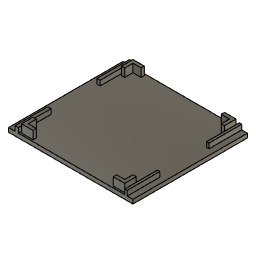
Batterystand V4 (Autodesk Fusion 360 design; units mm, degrees)
Autodesk Fusion 360 part; units mm, degrees
sketch "Sketch2" plane through (0, 0, 0) normal (0, 0, 1) x (1, 0, 0)
  line L0 (0, 0) -> (76, 0)
  line L1 (76, 0) -> (76, 70)
  line L2 (76, 70) -> (0, 70)
  line L3 (0, 70) -> (0, 0)
  dimension "d20" = 76
  dimension "d21" = 70
  constraint horizontal L0
  constraint vertical L1
  constraint horizontal L2
  constraint vertical L3
  constraint coincident L0.start L3.end
  measures "d20" distance of L0.start L0.end
  measures "d21" distance of L0.start L2.end
extrude "Extrude1" add sketch "Sketch2" along normal blind 2.9
sketch "Sketch3" plane through (0, 0, 2.9) normal (0, 0, 1) x (-1, 0, 0)
  line L0 (0, -70) -> (0, 0)
  line L1 (0, 0) -> (-76, 0)
  line L2 (-76, 0) -> (-76, -70)
  line L3 (-76, -70) -> (0, -70)
  line L4 (0, -70) -> (-7, -70)
  line L5 (-7, -70) -> (-7, -69)
  line L6 (-7, -69) -> (-14, -69)
  line L7 (-14, -69) -> (-14, -67)
  line L8 (-14, -67) -> (-9, -67)
  line L9 (-9, -67) -> (-9, -62)
  line L10 (-9, -62) -> (-7, -62)
  line L11 (-7, -62) -> (-7, -69)
  line L12 (-9, -67) -> (-68, -67)
  line L13 (-68, -67) -> (-63, -67)
  line L14 (-63, -67) -> (-63, -69)
  line L15 (-63, -69) -> (-70, -69)
  line L16 (-70, -69) -> (-70, -62)
  line L17 (-70, -62) -> (-68, -62)
  line L18 (-68, -62) -> (-68, -67)
  line L19 (-68, -67) -> (-68, -3)
  line L20 (-68, -3) -> (-63, -3)
  line L21 (-63, -3) -> (-63, -1)
  line L22 (-63, -1) -> (-70, -1)
  line L23 (-70, -1) -> (-70, -8)
  line L24 (-70, -8) -> (-68, -8)
  line L25 (-68, -3) -> (-68, -8)
  line L26 (-9, -67) -> (-9, -3)
  line L27 (-9, -3) -> (-14, -3)
  line L28 (-14, -3) -> (-14, -1)
  line L29 (-14, -1) -> (-7, -1)
  line L30 (-7, -1) -> (-7, -8)
  line L31 (-7, -8) -> (-9, -8)
  line L32 (-9, -3) -> (-9, -8)
  dimension "d24" = 7
  dimension "d25" = 1
  dimension "d26" = 7
  dimension "d27" = 2
  dimension "d28" = 5
  dimension "d29" = 5
  dimension "d30" = 2
  dimension "d31" = 59
  dimension "d32" = 5
  dimension "d33" = 2
  dimension "d34" = 64
  dimension "d35" = 5
  dimension "d36" = 2
  dimension "d37" = 7
  dimension "d38" = 7
  dimension "d39" = 2
  dimension "d40" = 64
  dimension "d41" = 5
  dimension "d42" = 2
  dimension "d43" = 7
  dimension "d44" = 7
  constraint coincident L0.start L3.end
  constraint perpendicular L0 L4
  constraint perpendicular L3 L5
  constraint perpendicular L5 L6
  constraint perpendicular L3 L7
  constraint perpendicular L7 L8
  constraint perpendicular L8 L9
  constraint perpendicular L9 L10
  constraint perpendicular L9 L12
  constraint parallel L12 L13
  constraint perpendicular L12 L14
  constraint perpendicular L14 L15
  constraint perpendicular L15 L16
  constraint perpendicular L14 L17
  constraint perpendicular L12 L19
  constraint perpendicular L18 L20
  constraint perpendicular L12 L21
  constraint perpendicular L21 L22
  constraint perpendicular L12 L23
  constraint perpendicular L23 L24
  constraint parallel L19 L25
  constraint perpendicular L8 L26
  constraint perpendicular L9 L27
  constraint perpendicular L1 L28
  constraint perpendicular L9 L29
  constraint perpendicular L29 L30
  constraint coincident L26 L31.end
  constraint perpendicular L26 L31
  measures "d24" distance of L0.start L4.end
  measures "d25" distance of L4.end L5.end
  measures "d26" distance of L5.end L6.end
  measures "d27" distance of L6.end L7.end
  measures "d28" distance of L7.end L8.end
  measures "d29" distance of L8.end L9.end
  measures "d30" distance of L9.end L10.end
  measures "d31" distance of L8.end L12.end
  measures "d32" distance of L12.end L13.end
  measures "d33" distance of L13.end L14.end
  measures "d34" distance of L12.end L19.end
  measures "d35" distance of L19.end L20.end
  measures "d36" distance of L20.end L21.end
  measures "d37" distance of L21.end L22.end
  measures "d38" distance of L22.end L23.end
  measures "d39" distance of L23.end L24.end
  measures "d40" distance of L8.end L26.end
  measures "d41" distance of L26.end L27.end
  measures "d42" distance of L27.end L28.end
  measures "d43" distance of L28.end L29.end
  measures "d44" distance of L29.end L30.end
extrude "Extrude2" add sketch "Sketch3" along normal blind 5 contours L6 L7 L8 L9 L10 L11 L12 L26 | L12 L13 L14 L15 L16 L17 L18 L19 | L19 L20 L21 L22 L23 L24 L25 | L26 L27 L28 L29 L30 L31 L32
extrude "Extrude3" cut 1 faces at (25.3333, 46.6667, 0) along direction (0, 0, 1) blind 1
sketch "Sketch4" plane through (0, 0, 2.9) normal (0, 0, 1) x (-1, 0, 0)
  line L0 (-14, -3) -> (-14, -1)
  line L1 (-14, -1) -> (-7, -1)
  line L2 (-7, -1) -> (-7, -8)
  line L3 (-7, -8) -> (-9, -8)
  line L4 (-9, -8) -> (-9, -3)
  line L5 (-9, -3) -> (-14, -3)
  line L6 (-9, -67) -> (-9, -62)
  line L7 (-9, -62) -> (-7, -62)
  line L8 (-7, -62) -> (-7, -69)
  line L9 (-7, -69) -> (-14, -69)
  line L10 (-14, -69) -> (-14, -67)
  line L11 (-14, -67) -> (-9, -67)
  line L12 (-63, -3) -> (-68, -3)
  line L13 (-68, -3) -> (-68, -8)
  line L14 (-68, -8) -> (-70, -8)
  line L15 (-70, -8) -> (-70, -1)
  line L16 (-70, -1) -> (-63, -1)
  line L17 (-63, -1) -> (-63, -3)
  line L18 (-63, -67) -> (-63, -69)
  line L19 (-63, -69) -> (-70, -69)
  line L20 (-70, -69) -> (-70, -62)
  line L21 (-70, -62) -> (-68, -62)
  line L22 (-68, -62) -> (-68, -67)
  line L23 (-68, -67) -> (-63, -67)
  line L24 (0, -70) -> (0, 0)
  line L25 (0, 0) -> (-76, 0)
  line L26 (-76, 0) -> (-76, -70)
  line L27 (-76, -70) -> (0, -70)
  line L28 (0, -70) -> (-4, -70)
  line L29 (-4, -70) -> (-6, -70)
  line L30 (-6, -70) -> (-6, -50)
  line L31 (-6, -50) -> (-4, -50)
  line L32 (-4, -50) -> (-4, -70)
  line L33 (-76, -70) -> (-72.5, -70)
  line L34 (-72.5, -70) -> (-71, -70)
  line L35 (-71, -70) -> (-71, -50)
  line L36 (-71, -50) -> (-72.5, -50)
  line L37 (-72.5, -50) -> (-72.5, -70)
  line L38 (0, -70) -> (0, -35)
  line L39 (0, -35) -> (-68, -35)
  line L40 (-4, -20) -> (-4, 0)
  line L41 (-4, 0) -> (-6, 0)
  line L42 (-6, 0) -> (-6, -20)
  line L43 (-6, -20) -> (-4, -20)
  line L44 (-71, 0) -> (-71, -20)
  line L45 (-72.5, 0) -> (-71, 0)
  line L46 (-72.5, -20) -> (-72.5, 0)
  line L47 (-71, -20) -> (-72.5, -20)
  dimension "d49" = 4
  dimension "d50" = 2
  dimension "d51" = 20
  dimension "d52" = 3.5
  dimension "d53" = 20
  dimension "d54" = 35
  constraint coincident L24.start L27.end
  constraint perpendicular L24 L28
  constraint horizontal L29
  constraint vertical L30
  constraint horizontal L31
  constraint vertical L32
  constraint coincident L26.end L27.start
  constraint perpendicular L26 L33
  constraint horizontal L34
  constraint vertical L35
  constraint horizontal L36
  constraint vertical L37
  constraint vertical L38
  constraint perpendicular L26 L39
  constraint symmetric L28.end L39 L40.end
  constraint symmetric L29.end L39 L41.end
  constraint symmetric L30.end L39 L42.end
  constraint symmetric L31.end L39 L40.start
  constraint symmetric L33.end L39 L45.start
  constraint symmetric L34.end L39 L44.start
  constraint symmetric L35.end L39 L44.end
  constraint symmetric L36.end L39 L46.start
  measures "d49" distance of L24.start L28.end
  measures "d50" distance of L28.end L29.end
  measures "d51" distance of L28.end L31.end
  measures "d52" distance of L26.end L33.end
  measures "d53" distance of L33.end L36.end
  measures "d54" distance of L24.start L38.end
extrude "Extrude4" add sketch "Sketch4" along normal blind 3 contours L27 L29 L30 L31 L32 | L25 L40 L41 L42 L43 | L27 L34 L35 L36 L37 | L25 L44 L45 L46 L47
sketch "Sketch5" plane through (0, 0, 1) normal (0, 0, -1) x (1, 0, 0)
  line L0 (0, 0) -> (0, -70)
  line L1 (0, -70) -> (76, -70)
  line L2 (76, -70) -> (76, 0)
  line L3 (76, 0) -> (0, 0)
  line L4 (0, 0) -> (76, 0)
  line L5 (76, 0) -> (76, -70)
  line L6 (76, -70) -> (0, -70)
  line L7 (0, -70) -> (0, 0)
  constraint horizontal L4
  constraint vertical L5
  constraint horizontal L6
  constraint vertical L7
  constraint coincident L1.end L2.start
  constraint coincident L0.start L3.end
extrude "Extrude5" add sketch "Sketch5" along normal blind 0.6
equation "d54 = ( 70 / 2 ) * 1 mm"
